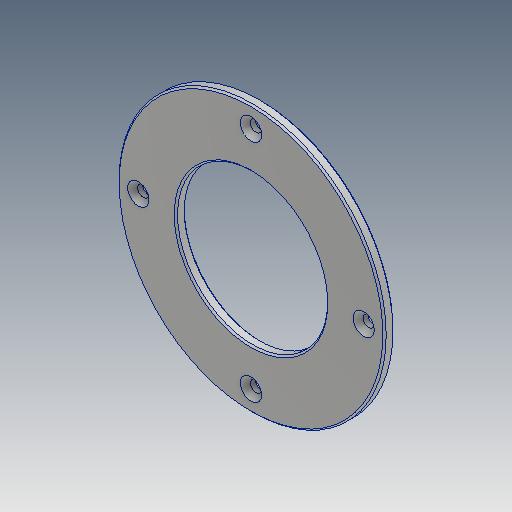
# Autodesk Inventor part: 200-10-ROCKER-BEARING-03
Saved by Autodesk Inventor 2018.2 (Build 222227000, 227)
## iProperties
Manager: feesmrt
Company: FRANC0R
Created: 2017-10-30
Part Number: 200-10-ROCKER-BEARING-03
Material: Aluminium 6061
Document SubType Name: Modeling
Designer: feesmrt
Density: 2.7 g/cm^3
Appearance: Aluminium - flach
Project: Rescue Robot
Cost Center: -
Description: Rocker Bearing Housing Cover Axle
Engineer: feesmrt
Authority: feesmrt
Stock Number: 200-10-ROCKER-BEARING-03
Author: feesmrt
Title: Rocker Bearing Housing Cover Axle
Subject: Rescue Robot
Revision Number: 1
Autodesk Inventor part; units mm, degrees
ref_plane "YZ Plane" through (0, 0, 0) normal (1, 0, 0) x (0, 1, 0)
ref_plane "XZ Plane" through (0, 0, 0) normal (0, 1, 0) x (-1, 0, 0)
ref_plane "XY Plane" through (0, 0, 0) normal (0, 0, 1) x (1, 0, 0)
derived "200-10-ROCKER-BEARING-01.ipt"
sketch "Skizze_RWDR" plane through (0, 0, 0) normal (1, 0, 0) x (0, 1, 0)
  line L0 (-32.5, -40) -> (-32.5, 40)
  line L1 (-32.5, 40) -> (-29.5, 40)
  line L2 (-29.5, -40) -> (-29.5, 40)
  line L3 (-32.5, -40) -> (-29.5, -40)
  line L4 (-29.5, 27.5) -> (-21.7, 27.5)
  line L5 (-21.2, -27) -> (-21.2, 27)
  line L6 (-29.5, -27.5) -> (-21.7, -27.5)
  arc A0 (-21.7, -27.5) -> (-21.2, -27) centre (-21.7, -27) ccw
  arc A1 (-21.2, 27) -> (-21.7, 27.5) centre (-21.7, 27) ccw
  line L7 (-21.2, 22.5) -> (-17.5, 22.5)
  line L8 (-21.2, -22.5) -> (-17.5, -22.5)
  line L9 (-17.5, 22.5) -> (-17.5, -22.5)
  point P0 (0, 0)
sketch "Skizze3" plane through (0, 0, 0) normal (1, 0, 0) x (0, 1, 0)
  line L0 (-32.5, -40) -> (-32.5, 40) construction
  line L1 (-29.5, -40) -> (-29.5, 40) construction
  line L2 (-32.5, 40) -> (-29.5, 40) construction
  line L3 (-32.5, -40) -> (-29.5, -40) construction
  line L4 (-32.5, 40) -> (-29.5, 40)
  line L5 (-29.5, 40) -> (-29.5, 22.5)
  line L6 (-32.5, 22.5) -> (-32.5, 40)
  line L7 (-32.5, 0) -> (-29.5, 0)
  line L8 (-32.5, 22.5) -> (-29.5, 22.5)
  line L9 (-21.2, 22.5) -> (-17.5, 22.5) construction
  point P0 (0, 0)
  constraints: 14 end point, 2 horizontal, 2 midpoint, 2 point on line, 1 horizontal alignment, 1 parallel, 1 perpendicular
revolve "Grundkoerper" add sketch "Skizze3" angle 360 about axis through (0, -32.5, 0) along (0, 1, 0)
sketch "Skizze4" plane through (0, -32.5, 0) normal (0, -1, 0) x (1, 0, 0)
  circle A0 centre (0, 0) radius 27.5 construction
  circle A1 centre (0, 0) radius 40 construction
  circle A2 centre (0, 0) radius 33.75 construction
  line L0 (0, 56) -> (0, -56) construction
  point P0 (0, 27.5)
  point P1 (0, 27.5)
  point P2 (0, 27.5)
  point P3 (0, -27.5)
  point P4 (0, -27.5)
  point P5 (0, -27.5)
  point P6 (0, 33.75)
  point P7 (-33.75, 0)
  point P8 (0, -33.75)
  point P9 (33.75, 0)
  dimension "d3" = 55
  dimension "d5" = 67.5
  dimension "d4" = 80
  dimension "d8" = 360
  constraints: 2 coincident, 2 vertical alignment, 11 other
  measures "d4" diameter of A1
hole "M3_Bohrung" at (0, -32.5, 33.75) at (-33.75, -32.5, 0) at (0, -32.5, -33.75) at (33.75, -32.5, 0) direction (0, 1, 0) diameter 3.4 end through all countersink diameter 6.4 countersink angle 90
chamfer "Fase_Allgemein" distance 0.5 angle 45 4 edges at (0, -32.5, -22.5) (0, -29.5, -22.5) (0, -32.5, -40) (0, -29.5, -40)
equation "\"d5\" = 0.5 * d4 + 0.5 * d3"
